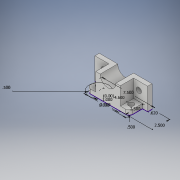
# Autodesk Inventor part: B
Saved by Autodesk Inventor 2018 (Build 220112000, 112)
## iProperties
Created: 2017-09-30
Part Number: B
Material: Generic
Document SubType Name: Modeling
Designer: Soichi
Density: 1 g/cm^3
Appearance: Default
Author: Soichi
Autodesk Inventor part; units mm, degrees
ref_plane "YZ Plane" through (0, 0, 0) normal (1, 0, 0) x (0, 1, 0)
ref_plane "XZ Plane" through (0, 0, 0) normal (0, 1, 0) x (-1, 0, 0)
ref_plane "XY Plane" through (0, 0, 0) normal (0, 0, 1) x (1, 0, 0)
sketch "Sketch1" plane through (0, 0, 0) normal (0, 0, 1) x (1, 0, 0)
  line L0 (-95.25, 15.748) -> (95.25, 15.748)
  line L1 (95.25, 15.748) -> (95.25, 0)
  line L2 (95.25, 0) -> (-95.25, 0)
  line L3 (-95.25, 0) -> (-95.25, 15.748)
  line L4 (-76.2, 0) -> (76.2, 0)
  line L5 (76.2, 0) -> (76.2, -35.052)
  line L6 (63.5, -47.752) -> (-63.5, -47.752)
  line L7 (-76.2, -35.052) -> (-76.2, 0)
  arc A0 (-76.2, -35.052) -> (-63.5, -47.752) centre (-63.5, -35.052) ccw
  arc A1 (63.5, -47.752) -> (76.2, -35.052) centre (63.5, -35.052) ccw
  line L8 (-58.42, -22.352) -> (58.42, -22.352) construction
  line L9 (-58.42, -22.352) -> (58.42, -22.352) construction
  line L10 (0, -22.352) -> (0, -47.752) construction
  line L11 (-44.45, 15.748) -> (44.45, 15.748)
  line L12 (44.45, 15.748) -> (44.45, -47.752)
  line L13 (44.45, -47.752) -> (-44.45, -47.752)
  line L14 (-44.45, -47.752) -> (-44.45, 15.748)
  point P0 (0, 0)
  point P1 (0, 0)
  point P2 (0, 15.748)
  dimension "d0" = 190.5
  dimension "d1" = 15.748
  dimension "d4" = 63.5
  dimension "d5" = 152.4
  dimension "d6" = 12.7
  dimension "d7" = 12.7
  dimension "d8" = 116.84
  dimension "d9" = 0
  dimension "d10" = 25.4
  dimension "d11" = 63.5
  dimension "d12" = 88.9
  constraints: 30 end point, 6 midpoint, 6 parallel, 5 horizontal, 4 point on circle, 4 tangent, 3 coincident, 3 perpendicular, 2 centre point, 1 collinear, 1 vertical
  measures "d0" distance of L0.start L0.end
  measures "d1" distance of L0.end L1.end
  measures "d4" distance between parallel lines of L6 L0
  measures "d5" distance between parallel lines of L7 L5
  measures "d6" radius of A0
  measures "d7" radius of A1
  measures "d8" distance of L8.start L8.end
  measures "d9" distance between parallel lines of L8 L9
  measures "d10" distance of L10.end L10.start
  measures "d11" distance of L11.end L12.end
  measures "d12" distance of L12.end L13.end
extrude "Extrusion1" add sketch "Sketch1" along normal blind 79.375 contours L0 L14 L2 L3 | L0 L12 L2 L14 | L0 L1 L2 L12 | L2 L12 L6 L14
extrude "Extrusion2" add sketch "Sketch1" along normal blind 15.748 contours L14 L6 A0 L7 L2 | L2 L12 L6 L14 | L2 L5 A1 L6 L12
sketch "Sketch2" plane through (-44.45, -47.752, 79.375) normal (0, -1, 0) x (1, 0, 0)
  line L0 (139.7, 0) -> (-50.8, 0) construction
  circle A0 centre (44.45, 0) radius 28.575
  line L1 (-19.05, 0) -> (107.95, 0) construction
  line L2 (0, 0) -> (88.9, 0) construction
  line L3 (-19.05, 0) -> (-19.05, -28.575) construction
  line L4 (44.45, 0) -> (44.45, -8.2892) construction
  circle A1 centre (-19.05, -28.575) radius 9.525
  circle A2 centre (107.95, -28.575) radius 9.525
  point P0 (44.45, -79.375)
  dimension "d17" = 57.15
  dimension "d18" = 127
  dimension "d23" = 28.575
  dimension "d24" = 19.05
  constraints: 6 end point, 3 centre point, 3 midpoint, 2 vertical, 1 coincident, 1 horizontal, 1 symmetric about line, 1 other
  measures "d17" diameter of A0
  measures "d18" distance of L1.start L1.end
  measures "d23" distance of L1.start L3.end
  measures "d24" diameter of A1
extrude "Extrusion3" cut sketch "Sketch2" against normal blind 63.5
hole "Hole1" at (-58.42, -22.352, 0) at (58.42, -22.352, 0) direction (0, 0, 1) diameter 19.05 end through all
body "Solid1"
